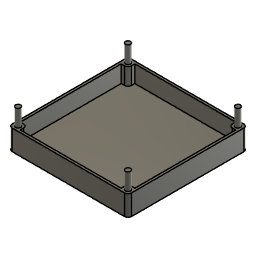
thermalkansi v2 (Autodesk Fusion 360 design; units mm, degrees)
Autodesk Fusion 360 part; units mm, degrees
sketch "Sketch1" plane through (0, 0, 0) normal (0, 1, 0) x (1, 0, 0)
  line L0 (0, 0) -> (-70, 0)
  line L1 (-70, 0) -> (-70, 70)
  line L2 (-70, 70) -> (0, 70)
  line L3 (0, 70) -> (0, 0)
  dimension "d1" = 70
  dimension "d2" = 70
  constraint horizontal L0
  constraint vertical L1
  constraint horizontal L2
  constraint vertical L3
  constraint coincident L0.start L3.end
  measures "d1" distance of L0.start L0.end
  measures "d2" distance of L0.start L2.end
extrude "Extrude1" add sketch "Sketch1" along normal blind 2
sketch "Sketch2" plane through (0, 2, 0) normal (0, 1, 0) x (-1, 0, 0)
  line L0 (0, -70) -> (70, -70)
  line L1 (70, -70) -> (70, 0)
  line L2 (70, 0) -> (0, 0)
  line L3 (0, 0) -> (0, -70)
  circle A0 centre (2.7499, -2.7499) radius 1.5
  line L4 (70, -70) -> (73.889, -70) construction
  line L5 (0, -70) -> (3.889, -70) construction
  circle A1 centre (67.2501, -67.2501) radius 1.5
  circle A2 centre (2.7499, -67.2501) radius 1.5
  circle A3 centre (67.2501, -2.7499) radius 1.5
  dimension "d5" = 3.889
  dimension "d6" = 3
  dimension "d7" = 3.889
  dimension "d9" = 3.889
  dimension "d11" = 3.889
  dimension "d12" = 3
  dimension "d13" = 3
  dimension "d14" = 3
  constraint horizontal L4
  constraint coincident L0.end L1.start
  constraint horizontal L5
  constraint coincident L0.start L3.end
  measures "d5" distance of L2.end A0.centre
  measures "d6" diameter of A0
  measures "d7" distance of L1.end A3.centre
  measures "d9" distance of L0.end A1.centre
  measures "d11" distance of L0.start A2.centre
  measures "d12" diameter of A1
  measures "d13" diameter of A2
  measures "d14" diameter of A3
extrude "Extrude2" add sketch "Sketch2" along normal blind 20 contours A0 | A1 | A2 | A3
fillet "Fillet1" radius 2 4 edges at (-70, 1, 0) (0, 1, 0) (0, 1, -70) (-70, 1, -70)
sketch "Sketch3" plane through (0, 2, 0) normal (0, 1, 0) x (-1, 0, 0)
  arc A0 (68, -70) -> (70, -68) centre (68, -68) ccw
  line L0 (70, -68) -> (70, -2)
  arc A1 (70, -2) -> (68, 0) centre (68, -2) ccw
  line L1 (68, 0) -> (2, 0)
  arc A2 (2, 0) -> (0, -2) centre (2, -2) ccw
  line L2 (0, -2) -> (0, -68)
  arc A3 (0, -68) -> (2, -70) centre (2, -68) ccw
  line L3 (2, -70) -> (68, -70)
  circle A4 centre (67.2501, -2.7499) radius 1.5
  circle A5 centre (67.2501, -67.2501) radius 1.5
  circle A6 centre (2.7499, -2.7499) radius 1.5
  circle A7 centre (2.7499, -67.2501) radius 1.5
  line L4 (0, 0) -> (70, 0)
  line L5 (70, 0) -> (70, -70)
  line L6 (70, -70) -> (0, -70)
  line L7 (0, -70) -> (0, 0)
  line L8 (68.0791, -66) -> (68, -66)
  line L9 (36, -1.414) -> (5.414, -1.414)
  line L10 (2, -5.414) -> (5.414, -5.414)
  line L11 (5.414, -5.414) -> (5.414, -1.414)
  line L12 (2, -5.414) -> (1.414, -5.414)
  line L13 (1.414, -15) -> (1.414, -5.414)
  line L14 (1.414, -15) -> (1.414, -64.586)
  line L15 (1.414, -64.586) -> (5.414, -64.586)
  line L16 (5.414, -64.586) -> (5.414, -68.586)
  line L17 (32, -68.586) -> (5.414, -68.586)
  line L18 (32, -68.586) -> (64.586, -68.586)
  line L19 (64.586, -68.586) -> (64.586, -64.586)
  line L20 (64.586, -64.586) -> (68.586, -64.586)
  line L21 (36, -1.414) -> (64.586, -1.414)
  line L22 (64.586, -1.414) -> (64.586, -5.414)
  line L23 (68.586, -24) -> (68.586, -5.414)
  line L24 (64.586, -5.414) -> (68.586, -5.414)
  line L25 (68.586, -24) -> (68.586, -64.586)
  line L26 (68, -66) -> (68, -65.951)
  dimension "d22" = 5.414
  dimension "d29" = 90
  constraint horizontal L4
  constraint vertical L5
  constraint horizontal L6
  constraint vertical L7
  constraint coincident L4.start L7.end
  constraint perpendicular L4 L13
  constraint perpendicular L12 L13
  constraint vertical L16
  constraint perpendicular L16 L17
  constraint perpendicular L8 L19
  constraint perpendicular L5 L20
  constraint perpendicular L5 L24
  constraint perpendicular L23 L24
  constraint perpendicular L20 L25
  constraint coincident A5 L8.start
  constraint coincident A5 L26.end
  measures "d22" distance of L1.end L10.start
  measures "d29" angle of L10 L11
extrude "Extrude3" add sketch "Sketch3" along normal blind 10 contours A0 L0 A1 L1 A2 L2 A3 L3 L4 L5 L6 L7
fillet "Fillet2" radius 2 2 edges at (-5.414, 7, -64.586) (-64.586, 7, -64.586)
fillet "Fillet3" radius 2 2 edges at (-64.586, 7, -5.414) (-5.414, 7, -5.414)
